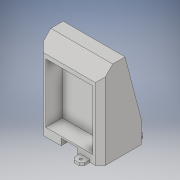
# Autodesk Inventor part: Speaker
Saved by Autodesk Inventor 2019.4 (Build 234330000, 330)
## iProperties
Created: 2020-04-11
Part Number: Speaker
Material: Типовые
Document SubType Name: Modeling
Designer: NoName
Density: 1 g/cm^3
Appearance: По умолчанию
Author: NoName
Autodesk Inventor part; units mm, degrees
ref_plane "YZ Plane" through (0, 0, 0) normal (1, 0, 0) x (0, 1, 0)
ref_plane "XZ Plane" through (0, 0, 0) normal (0, 1, 0) x (-1, 0, 0)
ref_plane "XY Plane" through (0, 0, 0) normal (0, 0, 1) x (1, 0, 0)
sketch "Эскиз1" plane through (0, 0, 0) normal (0, 1, 0) x (-1, 0, 0)
  line L0 (37.5, -50) -> (-37.5, -50)
  line L1 (-37.5, -50) -> (-37.5, 0)
  line L2 (-37.5, 0) -> (37.5, 0)
  line L3 (37.5, 0) -> (37.5, -50)
  point P0 (0, 0)
  point P1 (0, 0)
  dimension "d0" = 75
  dimension "d1" = 50
  constraints: 8 end point, 2 parallel, 1 coincident, 1 horizontal, 1 midpoint, 1 perpendicular
  measures "d0" distance between parallel lines of L1 L3
  measures "d1" distance between parallel lines of L2 L0
extrude "Выдавливание1" add sketch "Эскиз1" along normal blind 10
sketch "Эскиз2" plane through (0, 10, 0) normal (0, 1, 0) x (1, 0, 0)
  line L0 (37.5, 50) -> (-37.5, 50) projected
  line L1 (-37.5, 50) -> (37.5, 50)
  line L2 (37.5, 50) -> (37.5, 0)
  line L3 (-37.5, 0) -> (-37.5, 50)
  line L4 (-37.5, 0) -> (-28.5, 0)
  line L5 (-28.5, 0) -> (-28.5, 20)
  line L6 (-28.5, 20) -> (28.5, 20)
  line L7 (28.5, 20) -> (28.5, 0)
  line L8 (-37.5, 0) -> (37.5, 0) construction
  line L9 (28.5, 0) -> (37.5, 0)
  point P0 (0, 0)
  point P1 (0, 20)
  point P2 (0, 0)
  dimension "d4" = 57
  dimension "d5" = 20
  constraints: 16 end point, 5 perpendicular, 2 horizontal, 2 midpoint, 1 parallel, 1 point on line, 1 vertical alignment
  measures "d4" distance of L5.end L6.end
  measures "d5" distance between parallel lines of L8 L6
extrude "Выдавливание2" add sketch "Эскиз2" along normal blind 72
sketch "Эскиз3" plane through (0, 82, 0) normal (0, 1, 0) x (1, 0, 0)
  line L0 (-37.5, 50) -> (-37.5, 0) projected
  line L1 (37.5, 50) -> (-37.5, 50) projected
  line L2 (-37.5, 0) -> (37.5, 0)
  line L3 (37.5, 0) -> (37.5, 50)
  line L4 (37.5, 50) -> (-37.5, 50)
  line L5 (-37.5, 50) -> (-37.5, 0)
  point P0 (0, 0)
  constraints: 8 end point, 2 parallel, 1 horizontal, 1 perpendicular
extrude "Выдавливание3" add sketch "Эскиз3" along normal blind 20
sketch "Эскиз4" plane through (37.5, 0, 0) normal (1, 0, 0) x (0, 0, -1)
  line L0 (0, 102) -> (50, 102) projected
  line L1 (30, 102) -> (50, 25)
  line L2 (50, 0) -> (50, 102) projected
  point P0 (0, 0)
  dimension "d10" = 30
  dimension "d11" = 25
  constraints: 2 end point, 2 point on line
  measures "d10" distance of L0.start L1.start
  measures "d11" distance of L2.start L1.end
extrude "Выдавливание4" cut sketch "Эскиз4" against normal through all
sketch "Эскиз5" plane through (37.5, 102, -30) normal (0, 0.2513984, -0.9678837) x (-1, 0, 0)
  circle A0 centre (37.5, -42.555) radius 36.5
  line L0 (75, -79.555) -> (0, -79.555) projected
  circle A1 centre (37.5, -42.555) radius 44.5
  point P0 (37.5, -91.1822)
  dimension "d14" = 73
  dimension "d15" = 37
  dimension "d16" = 89
  constraints: 2 centre point, 1 coincident, 1 vertical alignment
  measures "d14" diameter of A0
  measures "d15" distance from line of L0 A0.centre
  measures "d16" diameter of A1
ref_plane "РабПлоскость2" through (37.5, 98.229, -15.4817) normal (0, 0.2513984, -0.9678837) x (-1, 0, 0)
sketch "Эскиз7" plane through (37.5, 98.229, -15.4817) normal (0, 0.2513984, -0.9678837) x (-1, 0, 0)
  point P0 (37.5, -91.1822)
sketch "Эскиз8" plane through (37.5, 98.229, -15.4817) normal (0, 0.2513984, -0.9678837) x (-1, 0, 0)
  circle A0 centre (37.5, -42.555) radius 44.5 projected
  circle A1 centre (37.5, -42.555) radius 14
  point P0 (37.5, -91.1822)
  dimension "d19" = 28
  constraints: 1 centre point, 1 coincident
  measures "d19" diameter of A1
loft "Лофт1" cut profiles "Эскиз8", "Эскиз5" contours A1 / A0
chamfer "Фаска1" distance 15 angle 45 1 edges at (0, 102, 0)
sketch "Эскиз9" plane through (37.5, 102, -30) normal (0, 0.2513984, -0.9678837) x (-1, 0, 0)
  line L0 (6, -8.2775) -> (69, -8.2775)
  line L1 (69, -8.2775) -> (69, -71.2775)
  line L2 (69, -71.2775) -> (6, -71.2775)
  line L3 (6, -71.2775) -> (6, -8.2775)
  line L4 (0, 0) -> (75, 0) projected
  line L5 (75, 0) -> (75, -79.555) projected
  point P0 (37.5, -91.1822)
  point P1 (37.5, -8.2775)
  point P2 (37.5, 0)
  point P3 (69, -39.7775)
  point P4 (75, -39.7775)
  dimension "d34" = 63
  constraints: 8 end point, 4 midpoint, 3 coincident, 2 parallel, 2 perpendicular, 1 horizontal, 1 horizontal alignment, 1 vertical alignment
  measures "d34" distance between parallel lines of L1 L3
hole "Отверстие1" at (31.5, 33.0117, -47.919) at (-31.5, 33.0117, -47.919) at (-31.5, 93.9883, -32.081) at (31.5, 93.9883, -32.081) direction (0, -0.2513984, 0.9678837) diameter 3 depth 16 tip angle 118
chamfer "Фаска2" distance 6 angle 45 2 edges at (-37.5, 43.5, 0) (37.5, 43.5, 0)
sketch "Эскиз10" plane through (0, 0, 0) normal (0, -1, 0) x (1, 0, 0)
  line L0 (-28.5, 0) -> (28.5, 0) projected
  line L1 (-37.5, -50) -> (37.5, -50) projected
  line L2 (-10, 0) -> (10, 0)
  line L3 (10, 0) -> (10, -50)
  line L4 (10, -50) -> (-10, -50)
  line L5 (-10, -50) -> (-10, 0)
  point P0 (0, 0)
  point P1 (0, 0)
  dimension "d39" = 20
  constraints: 8 end point, 2 midpoint, 2 parallel, 2 point on line, 1 horizontal, 1 perpendicular
  measures "d39" distance between parallel lines of L3 L5
extrude "Выдавливание5" cut sketch "Эскиз10" against normal blind 8
sketch "Эскиз11" plane through (0, 0, 0) normal (0, -1, 0) x (1, 0, 0)
  line L0 (10, -50) -> (37.5, -50) projected
  line L1 (32, -50) -> (20, -50)
  line L2 (20, -50) -> (20, -60)
  line L3 (20, -60) -> (32, -60)
  line L4 (32, -60) -> (32, -50)
  line L5 (-37.5, -50) -> (37.5, -50) projected
  line L6 (0, -50) -> (0, 0)
  line L7 (-10, -50) -> (-37.5, -50)
  line L8 (-32, -50) -> (-20, -50)
  line L9 (-20, -50) -> (-20, -60)
  line L10 (-20, -60) -> (-32, -60)
  line L11 (-32, -60) -> (-32, -50)
  line L12 (31.5, 0) -> (10, 0) projected
  line L13 (25, 0) -> (13, 0)
  line L14 (13, 0) -> (13, 10)
  line L15 (13, 10) -> (25, 10)
  line L16 (25, 10) -> (25, 0)
  line L17 (10, 0) -> (10, -50) projected
  dimension "d42" = 12
  dimension "d43" = 10
  dimension "d44" = 40
  dimension "d45" = 12
  dimension "d46" = 10
  dimension "d47" = 3
  constraints: 28 end point, 5 symmetric about line, 4 parallel, 3 point on line, 2 horizontal, 2 perpendicular, 1 midpoint, 1 vertical
  measures "d42" distance between parallel lines of L4 L2
  measures "d43" distance between parallel lines of L0 L3
  measures "d44" distance between parallel lines of L2 L9
  measures "d45" distance between parallel lines of L16 L14
  measures "d46" distance of L15.end L13.start
  measures "d47" distance between parallel lines of L14 L17
extrude "Выдавливание6" add sketch "Эскиз11" against normal blind 3
chamfer "Фаска3" distance 3 angle 45 6 edges at (20, 1.5, -60) (32, 1.5, -60) (-32, 1.5, -60) (-20, 1.5, -60) (25, 1.5, 10) (13, 1.5, 10)
sketch "Эскиз12" plane through (0, 0, 0) normal (0, -1, 0) x (1, 0, 0)
  line L0 (10, -50) -> (20, -50) projected
  line L1 (-10, -50) -> (-10, 0) projected
  line L2 (22, 10) -> (16, 10) projected
  point P0 (0, 0)
  point P1 (26, -55)
  point P2 (-26, -55)
  point P3 (19, 5)
  point P4 (19, 10)
  dimension "d60" = 52
  dimension "d61" = 60
  dimension "d62" = 5
  dimension "d63" = 16
  constraints: 1 horizontal alignment, 1 midpoint, 1 vertical alignment
  measures "d60" distance of point (26, -55) point (-26, -55)
  measures "d61" vertical distance of point (26, -55) point (19, 5)
  measures "d62" distance from line of L0 point (26, -55)
  measures "d63" distance from line of point (-26, -55) L1
hole "Отверстие2" at (26, 0, -55) at (-26, 0, -55) at (19, 0, 5) direction (0, 1, 0) diameter 3.2 depth 16 tip angle 118
sketch "Эскиз13" plane through (-37.5, 0, -50) normal (-1, 0, 0) x (0, 0, 1)
  circle A0 centre (18.2655, 63.5) radius 2.5
  line L0 (20, 102) -> (0, 25) projected
  point P0 (50, 0)
  point P1 (10, 63.5)
  dimension "d64" = 5
  dimension "d65" = 8
  constraints: 1 centre point, 1 horizontal alignment, 1 midpoint
  measures "d64" diameter of A0
  measures "d65" distance from line of L0 A0.centre
extrude "Выдавливание7" cut sketch "Эскиз13" against normal blind 20
